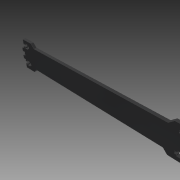
# Autodesk Inventor part: webcam_back_holder
Saved by Autodesk Inventor 2014 (Build 180170000, 170)
## iProperties
Created: 2014-01-22
Part Number: webcam_back_holder
Material: Generic
Document SubType Name: Modeling
Designer: buben
Density: 1 g/cm^3
Appearance: Anodized - Dark Gray
Author: buben
Autodesk Inventor part; units mm, degrees
ref_plane "YZ Plane" through (0, 0, 0) normal (1, 0, 0) x (0, 1, 0)
ref_plane "XZ Plane" through (0, 0, 0) normal (0, 1, 0) x (-1, 0, 0)
ref_plane "XY Plane" through (0, 0, 0) normal (0, 0, 1) x (1, 0, 0)
sketch "Sketch1" plane through (0, 0, 0) normal (0, 1, 0) x (-1, 0, 0)
  line L0 (0, 0) -> (347, 0)
  line L1 (347, 0) -> (347, 60)
  line L2 (347, 60) -> (0, 60)
  line L3 (0, 60) -> (0, 0)
  dimension "d0" = 60
  dimension "d1" = 347
  constraints: 8 end point, 2 parallel, 1 horizontal, 1 perpendicular
  measures "d0" distance of L2.end L0.start
  measures "d1" distance of L0.start L0.end
extrude "Extrusion1" add sketch "Sketch1" along normal blind 6
sketch "Sketch2" plane through (0, 6, 0) normal (0, 1, 0) x (1, 0, 0)
  line L0 (-347, 0) -> (-347, -60) projected
  line L1 (0, -60) -> (0, 0) projected
  line L2 (-347, -18) -> (-351, -18)
  line L3 (-353, -20) -> (-353, -24)
  line L4 (-351, -26) -> (-347, -26)
  line L5 (-347, -26) -> (-347, -18)
  line L6 (0, -18) -> (4, -18)
  line L7 (6, -20) -> (6, -24)
  line L8 (4, -26) -> (0, -26)
  line L9 (0, -26) -> (0, -18)
  arc A0 (-351, -18) -> (-353, -20) centre (-351, -20) ccw
  arc A1 (-353, -24) -> (-351, -26) centre (-351, -24) ccw
  arc A2 (6, -20) -> (4, -18) centre (4, -20) ccw
  arc A3 (4, -26) -> (6, -24) centre (4, -24) ccw
  line L10 (-347, -34) -> (-351, -34)
  line L11 (-353, -36) -> (-353, -40)
  line L12 (-351, -42) -> (-347, -42)
  line L13 (-347, -42) -> (-347, -34)
  line L14 (0, -34) -> (4, -34)
  line L15 (6, -36) -> (6, -40)
  line L16 (4, -42) -> (0, -42)
  line L17 (0, -42) -> (0, -34)
  arc A4 (-351, -34) -> (-353, -36) centre (-351, -36) ccw
  arc A5 (-353, -40) -> (-351, -42) centre (-351, -40) ccw
  arc A6 (6, -36) -> (4, -34) centre (4, -36) ccw
  arc A7 (4, -42) -> (6, -40) centre (4, -40) ccw
  line L18 (-349, -26) -> (-349, -34) construction
  point P0 (-349, -30)
  point P1 (-347, -30)
  dimension "d4" = 2
  dimension "d5" = 8
  dimension "d6" = 6
  dimension "d7" = 6
  dimension "d9" = 2
  dimension "d10" = 8
  dimension "d11" = 8
  constraints: 34 end point, 16 point on circle, 16 tangent, 8 centre point, 8 parallel, 6 collinear, 6 equal radius, 4 horizontal, 4 midpoint, 4 perpendicular, 4 point on line, 1 horizontal alignment
  measures "d4" radius of A0
  measures "d5" distance between parallel lines of L4 L2
  measures "d6" distance between parallel lines of L0 L3
  measures "d7" distance between parallel lines of L1 L7
  measures "d9" radius of A4
  measures "d10" distance between parallel lines of L12 L10
  measures "d11" distance of L18.start L18.end
extrude "Extrusion2" add sketch "Sketch2" against normal blind 6
sketch "Sketch3" plane through (0, 6, 0) normal (0, 1, 0) x (1, 0, 0)
  line L0 (0, 0) -> (-347, 0) projected
  line L1 (-347, 0) -> (-347, -18) projected
  line L2 (-347, -60) -> (0, -60) projected
  line L3 (-330.7, -9.75) -> (-330.7, -14.25)
  line L4 (-347, -14.25) -> (-347, -9.75)
  line L5 (-342, -7.25) -> (-334.7, -7.25)
  line L6 (-334.7, -16.75) -> (-342, -16.75)
  line L7 (-347, -9.75) -> (-342, -9.75)
  line L8 (-334.7, -9.75) -> (-330.7, -9.75)
  line L9 (-330.7, -14.25) -> (-334.7, -14.25)
  line L10 (-342, -14.25) -> (-347, -14.25)
  line L11 (-342, -16.75) -> (-342, -14.25)
  line L12 (-342, -9.75) -> (-342, -7.25)
  line L13 (-334.7, -7.25) -> (-334.7, -9.75)
  line L14 (-334.7, -14.25) -> (-334.7, -16.75)
  line L15 (-330.7, -45.75) -> (-330.7, -50.25)
  line L16 (-347, -50.25) -> (-347, -45.75)
  line L17 (-342, -43.25) -> (-334.7, -43.25)
  line L18 (-334.7, -52.75) -> (-342, -52.75)
  line L19 (-347, -45.75) -> (-342, -45.75)
  line L20 (-334.7, -45.75) -> (-330.7, -45.75)
  line L21 (-330.7, -50.25) -> (-334.7, -50.25)
  line L22 (-342, -50.25) -> (-347, -50.25)
  line L23 (-342, -52.75) -> (-342, -50.25)
  line L24 (-342, -45.75) -> (-342, -43.25)
  line L25 (-334.7, -43.25) -> (-334.7, -45.75)
  line L26 (-334.7, -50.25) -> (-334.7, -52.75)
  line L27 (-173.5, -60) -> (-173.5, 0) construction
  line L28 (-16.3, -9.75) -> (-16.3, -14.25)
  line L29 (0, -14.25) -> (0, -9.75)
  line L30 (-5, -7.25) -> (-12.3, -7.25)
  line L31 (-12.3, -16.75) -> (-5, -16.75)
  line L32 (0, -9.75) -> (-5, -9.75)
  line L33 (-12.3, -9.75) -> (-16.3, -9.75)
  line L34 (-16.3, -14.25) -> (-12.3, -14.25)
  line L35 (-5, -14.25) -> (0, -14.25)
  line L36 (-5, -16.75) -> (-5, -14.25)
  line L37 (-5, -9.75) -> (-5, -7.25)
  line L38 (-12.3, -7.25) -> (-12.3, -9.75)
  line L39 (-12.3, -14.25) -> (-12.3, -16.75)
  line L40 (-16.3, -50.25) -> (-12.3, -50.25)
  line L41 (-16.3, -45.75) -> (-16.3, -50.25)
  line L42 (-12.3, -45.75) -> (-16.3, -45.75)
  line L43 (-12.3, -43.25) -> (-12.3, -45.75)
  line L44 (-12.3, -50.25) -> (-12.3, -52.75)
  line L45 (-5, -43.25) -> (-12.3, -43.25)
  line L46 (-12.3, -52.75) -> (-5, -52.75)
  line L47 (-5, -52.75) -> (-5, -50.25)
  line L48 (-5, -45.75) -> (-5, -43.25)
  line L49 (0, -45.75) -> (-5, -45.75)
  line L50 (-5, -50.25) -> (0, -50.25)
  line L51 (0, -50.25) -> (0, -45.75)
  point P0 (-347, -42)
  point P1 (-330.7, -12)
  point P2 (-330.7, -48)
  point P3 (-16.3, -12)
  point P4 (-16.3, -48)
  dimension "d14" = 4.5
  dimension "d15" = 2.5
  dimension "d16" = 2.5
  dimension "d17" = 5
  dimension "d18" = 4
  dimension "d19" = 7.3
  dimension "d20" = 4.5
  dimension "d21" = 2.5
  dimension "d22" = 2.5
  dimension "d23" = 5
  dimension "d24" = 4
  dimension "d25" = 7.3
  dimension "d26" = 6
  dimension "d27" = 6
  constraints: 98 end point, 26 symmetric about line, 20 parallel, 10 collinear, 8 perpendicular, 6 horizontal, 4 midpoint
  measures "d14" distance of L3.start L3.end
  measures "d15" distance of L5.end L8.start
  measures "d16" distance of L9.end L6.start
  measures "d17" distance of L4.end L7.end
  measures "d18" distance of L8.start L3.start
  measures "d19" distance of L5.start L5.end
  measures "d20" distance of L15.start L21.start
  measures "d21" distance of L25.start L20.start
  measures "d22" distance of L21.end L26.end
  measures "d23" distance of L19.start L24.start
  measures "d24" distance of L20.start L15.start
  measures "d25" distance of L17.start L25.start
  measures "d26" vertical distance of point (-330.7, -12) L1.end
  measures "d27" vertical distance of point (-330.7, -48) point (-347, -42)
extrude "Extrusion3" cut sketch "Sketch3" against normal blind 6
sketch "Sketch4" plane through (0, 6, 0) normal (0, 1, 0) x (1, 0, 0)
  line L0 (0, 0) -> (-347, 0) projected
  line L1 (-347, -60) -> (0, -60) projected
  line L2 (-5, -7.25) -> (-5, -9.75) projected
  line L3 (-322, 0) -> (-314, -8)
  line L4 (-314, -8) -> (-33, -8)
  line L5 (-33, -8) -> (-25, 0)
  line L6 (-322, -60) -> (-314, -52)
  line L7 (-314, -52) -> (-33, -52)
  line L8 (-33, -52) -> (-25, -60)
  dimension "d30" = 45
  dimension "d31" = 25
  dimension "d32" = 25
  dimension "d33" = 8
  dimension "d34" = 8
  constraints: 12 end point, 4 point on line, 3 perpendicular, 2 parallel, 2 vertical alignment
  measures "d30" angle of L0 L3
  measures "d31" distance of L0.end L3.start
  measures "d32" distance of L0.start L5.end
  measures "d33" distance between parallel lines of L0 L4
  measures "d34" distance between parallel lines of L1 L7
extrude "Extrusion4" cut sketch "Sketch4" against normal blind 6
equation "\"d16\" = d15"
equation "\"d22\" = d21"
equation "\"d27\" = d26"
equation "\"d34\" = d33"
body "Solid1"
